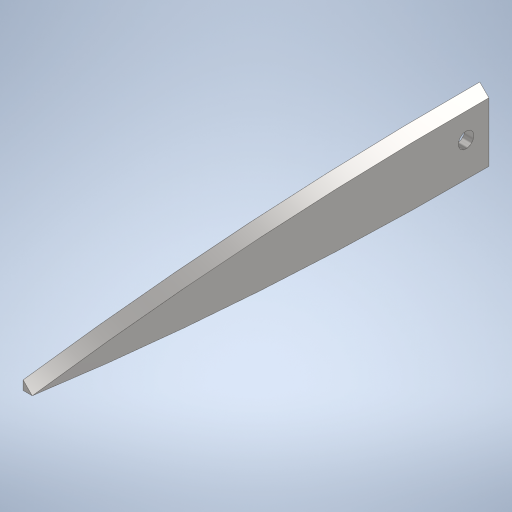
# Autodesk Inventor part: scissor
Saved by Autodesk Inventor 2024 (Build 280153000, 153)
## iProperties
Created: 2024-10-12
Part Number: scissor
Material: ステンレス鋼
Document SubType Name: Modeling
Designer: 1412z
Density: 8 g/cm^3
Appearance: 半つや出し
Author: 1412z
Autodesk Inventor part; units mm, degrees
ref_plane "YZ Plane" through (0, 0, 0) normal (1, 0, 0) x (0, 1, 0)
ref_plane "XZ Plane" through (0, 0, 0) normal (0, 1, 0) x (-1, 0, 0)
ref_plane "XY Plane" through (0, 0, 0) normal (0, 0, 1) x (1, 0, 0)
sketch "スケッチ1" plane through (0, 0, 0) normal (1, 0, 0) x (0, 1, 0)
  line L0 (0, 0) -> (15, 0)
  line L1 (7.5, 0) -> (7.5, 100)
  arc A0 (6.5, 100) -> (0, 0) centre (699.9841, 4.7123) ccw
  arc A1 (15, 0) -> (8.5, 100) centre (-684.9841, 4.7123) ccw
  line L2 (6.5, 100) -> (8.5, 100)
  dimension "d0" = 15
  dimension "d1" = 100
  dimension "d3" = 700
  dimension "d4" = 700
  constraints: 6 end point, 4 point on circle, 2 centre point, 2 horizontal, 1 midpoint, 1 vertical
  measures "d0" distance of L0.start L0.end
  measures "d1" distance of L1.start L1.end
  measures "d3" radius of A0
  measures "d4" radius of A1
extrude "押し出し1" add sketch "スケッチ1" against normal blind 2
chamfer "面取り1" distance 2 angle 45 1 edges at (0, 13.5418, 50.1165)
sketch "スケッチ2" plane through (0, 0, 0) normal (1, 0, 0) x (0, 0, -1)
  circle A0 centre (-5, 7.5) radius 1.7
  point P0 (0, 0)
  dimension "d10" = 3.4
  constraints: 1 centre point
  measures "d10" diameter of A0
extrude "押し出し2" cut sketch "スケッチ2" against normal blind 2
